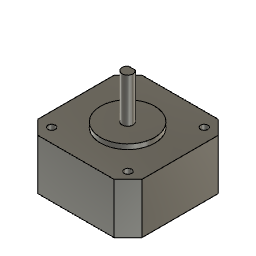
NEMA 17 Stepper Motor 42x42x20 v1 (Autodesk Fusion 360 design; units mm, degrees)
Autodesk Fusion 360 part; units mm, degrees
sketch "Sketch1" plane through (0, 0, 0) normal (0, 0, 1) x (1, 0, 0)
  line L0 (0, 0) -> (42.3, 0)
  line L1 (42.3, 0) -> (42.3, 42.3)
  line L2 (42.3, 42.3) -> (0, 42.3)
  line L3 (0, 42.3) -> (0, 0)
  line L4 (0, 0) -> (5.65, 0)
  line L5 (42.3, 5.65) -> (36.65, 0)
  line L6 (42.3, 5.65) -> (34.3097, 5.65) construction
  line L7 (5.65, 0) -> (0, 5.65)
  circle A0 centre (5.65, 5.65) radius 1.5
  circle A1 centre (36.6414, 5.65) radius 1.5
  circle A2 centre (5.65, 36.65) radius 1.5
  circle A3 centre (36.65, 36.65) radius 1.5
  line L8 (0, 36.65) -> (5.65, 42.3)
  line L9 (36.65, 42.3) -> (42.3, 36.65)
  dimension "d1" = 42.3
  dimension "d2" = 42.3
  dimension "d3" = 5.65
  dimension "d4" = 5.65
  dimension "d5" = 45
  dimension "d6" = 3
  dimension "d7" = 3
  dimension "d8" = 3
  dimension "d9" = 3
  constraint horizontal L0
  constraint vertical L1
  constraint horizontal L2
  constraint vertical L3
  constraint coincident L0.start L3.end
  constraint perpendicular L3 L4
  constraint coincident L3 L7.end
  constraint coincident L1 L5.start
  constraint horizontal L6
  constraint coincident L0 L5.end
  constraint coincident L2 L8.end
  constraint coincident L2 L9.start
  constraint coincident L3 L8.start
  constraint coincident L1 L9.end
  constraint coincident L6 A1.centre
  constraint perpendicular L8 L9
  measures "d1" distance of L0.start L0.end
  measures "d2" distance of L0.start L2.end
  measures "d3" distance of L0.start L4.end
  measures "d4" distance of L4.end A0.centre
  measures "d5" angle of L5 L6
  measures "d6" diameter of A0
  measures "d7" diameter of A1
  measures "d8" diameter of A2
  measures "d9" diameter of A3
extrude "Extrude1" add sketch "Sketch1" against normal blind 20.5 contours L0 L1 L2 L3 L5 L7 L8 L9
move_body "Move1" bodies 1 to x (1, 0, 0) y (0, 1, 0) z (0, 0, 1) at (0, 0, 20.5)
sketch "Sketch2" plane through (0, 0, 0) normal (0, 0, 1) x (1, 0, 0)
  circle A0 centre (21.15, 21) radius 11
  circle A1 centre (21.15, 21) radius 2.25
  line L0 (21.15, 23.25) -> (21.15, 22.75)
  line L1 (21.15, 22.75) -> (22.5642, 22.75)
  line L2 (21.15, 22.75) -> (19.7358, 22.75)
  dimension "d13" = 22
  dimension "d14" = 4.5
  dimension "d15" = 0.5
  constraint concentric A0 A1
  constraint coincident A1 L0.start
  constraint coincident A1 L1.end
  constraint coincident A1 L2.end
  measures "d13" diameter of A0
  measures "d14" diameter of A1
  measures "d15" distance of L0.start L0.end
extrude "Extrude2" add sketch "Sketch2" along normal blind 22.5 contours A0 | A1 L1 L2 | A1 L0 L1 | A1 L0 L2
extrude "Extrude3" add sketch "Sketch2" along normal blind 23 contours A1 L1 L2 | A1 L0 L1 | A1 L0 L2
extrude "Extrude4" add sketch "Sketch2" along normal blind 40.5 contours A1 L1 L2
